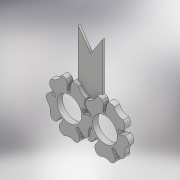
# Autodesk Inventor part: RosaV2
Saved by Autodesk Inventor 2017 (Build 210142000, 142)
## iProperties
Created: 2018-06-14
Part Number: RosaV2
Material: Generic
Document SubType Name: Modeling
Designer: Carolina Lema
Density: 1 g/cm^3
Appearance: Default
Author: Carolina Lema
Autodesk Inventor part; units mm, degrees
ref_plane "YZ Plane" through (0, 0, 0) normal (1, 0, 0) x (0, 1, 0)
ref_plane "XZ Plane" through (0, 0, 0) normal (0, 1, 0) x (-1, 0, 0)
ref_plane "XY Plane" through (0, 0, 0) normal (0, 0, 1) x (1, 0, 0)
sketch "Sketch1" plane through (0, 0, 0) normal (0, 1, 0) x (-1, 0, 0)
  arc A0 (-50.2935, -141.9625) -> (-50.5085, -138.2118) centre (-57.4787, -140.493) ccw
  arc A1 (-49.4604, -134.8668) -> (-50.5085, -138.2118) centre (-45.5145, -137.94) ccw
  arc A2 (-52.2706, -141.9093) -> (-53.5294, -134.3132) centre (-66.0628, -140.2926) ccw
  arc A3 (-60.8507, -147.4866) -> (-64.2809, -146.6761) centre (-66.0428, -161.7965) ccw
  circle A4 centre (-51.5636, -152.3854) radius 9
  arc A5 (-45.2271, -160.758) -> (-42.1345, -164.9104) centre (-15.6123, -141.9291) ccw
  arc A6 (-38.966, -164.9101) -> (-37.6707, -160.6686) centre (-43.0606, -161.3412) ccw
  arc A7 (-44.5421, -165.2935) -> (-46.8275, -161.7567) centre (-172.1244, -245.2288) ccw
  arc A8 (-37.8657, -145.4277) -> (-38.2191, -140.1494) centre (-41.6996, -143.0334) ccw
  arc A9 (-45.6096, -134.3885) -> (-38.2191, -140.1494) centre (-36.6467, -130.5112) ccw
  arc A10 (-36.1368, -156.274) -> (-37.6707, -160.6686) centre (-32.4682, -160.0194) ccw
  arc A11 (-36.1368, -156.274) -> (-34.6048, -152.385) centre (-42.1305, -151.6666) ccw
  arc A12 (-41.3682, -149.8747) -> (-38.503, -148.5121) centre (-47.6774, -132.9147) ccw
  arc A13 (-41.9398, -148.1863) -> (-37.8657, -145.4277) centre (-47.8277, -135.103) ccw
  arc A14 (-34.6048, -152.385) -> (-38.503, -148.5121) centre (-40.8573, -154.78) ccw
  arc A15 (-63.8657, -139.5775) -> (-58.174, -134.8668) centre (-65.1246, -132.2626) ccw
  arc A16 (-53.5294, -134.3132) -> (-58.174, -134.8668) centre (-55.4761, -137.7415) ccw
  arc A17 (-45.6096, -134.3885) -> (-49.4604, -134.8668) centre (-47.2959, -136.5525) ccw
  line L0 (-46.3394, -171.0352) -> (-46.3407, -171.0345)
  arc A18 (-48.8902, -170.6862) -> (-44.9412, -169.507) centre (-47.5666, -167.9168) ccw
  arc A19 (-65.6657, -161.3497) -> (-62.9245, -164.9101) centre (-62.7518, -161.9418) ccw
  arc A20 (-62.9245, -164.9101) -> (-58.2423, -160.4876) centre (-68.2851, -154.5449) ccw
  arc A21 (-56.5584, -161.6213) -> (-58.6246, -165.2834) centre (21.5695, -208.1162) ccw
  arc A22 (-58.6246, -165.2834) -> (-59.26, -166.6979) centre (-55.3426, -167.6077) ccw
  arc A23 (-59.26, -166.6979) -> (-53.816, -170.3276) centre (-55.8552, -167.4887) ccw
  arc A24 (-48.8902, -170.6862) -> (-53.816, -170.3276) centre (-51.7693, -176.2225) ccw
  arc A25 (-65.6657, -161.3497) -> (-67.4979, -155.3741) centre (-72.0774, -160.047) ccw
  arc A26 (-61.8781, -150.4206) -> (-66.2243, -148.9882) centre (-82.2432, -204.906) ccw
  arc A27 (-42.1345, -164.9104) -> (-38.966, -164.9101) centre (-40.5505, -161.8463) ccw
  arc A28 (-44.9412, -169.507) -> (-44.5421, -165.2935) centre (-48.2055, -167.0721) ccw
  arc A29 (-76.2935, -141.9625) -> (-76.5085, -138.2118) centre (-83.4787, -140.493) ccw
  arc A30 (-75.4604, -134.8668) -> (-76.5085, -138.2118) centre (-71.5145, -137.94) ccw
  arc A31 (-78.2706, -141.9093) -> (-79.5294, -134.3132) centre (-92.0628, -140.2926) ccw
  arc A32 (-86.8507, -147.4866) -> (-90.2809, -146.6761) centre (-92.0428, -161.7965) ccw
  circle A33 centre (-77.5636, -152.3854) radius 9
  arc A34 (-71.2271, -160.758) -> (-68.1345, -164.9104) centre (-41.6123, -141.9291) ccw
  arc A35 (-70.5421, -165.2935) -> (-72.8275, -161.7567) centre (-198.1244, -245.2288) ccw
  arc A36 (-63.8657, -145.4277) -> (-64.2191, -140.1494) centre (-67.6996, -143.0334) ccw
  arc A37 (-71.6096, -134.3885) -> (-64.2191, -140.1494) centre (-62.6467, -130.5112) ccw
  arc A38 (-67.9398, -148.1863) -> (-63.8657, -145.4277) centre (-73.8277, -135.103) ccw
  arc A39 (-90.7671, -139.6764) -> (-84.174, -134.8668) centre (-91.1246, -132.2626) ccw
  arc A40 (-79.5294, -134.3132) -> (-84.174, -134.8668) centre (-81.4761, -137.7415) ccw
  arc A41 (-71.6096, -134.3885) -> (-75.4604, -134.8668) centre (-73.2959, -136.5525) ccw
  line L1 (-72.3394, -171.0352) -> (-72.3407, -171.0345)
  arc A42 (-74.8902, -170.6862) -> (-70.9412, -169.507) centre (-73.5666, -167.9168) ccw
  arc A43 (-91.6657, -161.3497) -> (-88.9245, -164.9101) centre (-88.7518, -161.9418) ccw
  arc A44 (-88.9245, -164.9101) -> (-84.2423, -160.4876) centre (-94.2851, -154.5449) ccw
  arc A45 (-82.5584, -161.6213) -> (-84.6246, -165.2834) centre (-4.4305, -208.1162) ccw
  arc A46 (-84.6246, -165.2834) -> (-85.26, -166.6979) centre (-81.3426, -167.6077) ccw
  arc A47 (-85.26, -166.6979) -> (-79.816, -170.3276) centre (-81.8552, -167.4887) ccw
  arc A48 (-74.8902, -170.6862) -> (-79.816, -170.3276) centre (-77.7693, -176.2225) ccw
  arc A49 (-91.6639, -144.9966) -> (-90.2809, -146.6761) centre (-87.4857, -142.9652) ccw
  arc A50 (-90.7671, -139.6764) -> (-91.6639, -144.9966) centre (-87.4857, -142.9652) ccw
  arc A51 (-91.6657, -161.3497) -> (-94.028, -154.908) centre (-98.0774, -160.047) ccw
  arc A52 (-92.2243, -148.9882) -> (-94.028, -154.908) centre (-90.5316, -152.7386) ccw
  arc A53 (-87.8781, -150.4206) -> (-92.2243, -148.9882) centre (-108.2432, -204.906) ccw
  arc A54 (-68.1345, -164.9104) -> (-64.966, -164.9101) centre (-66.5505, -161.8463) ccw
  arc A55 (-70.9412, -169.507) -> (-70.5421, -165.2935) centre (-74.2055, -167.0721) ccw
  arc A56 (-66.2243, -148.9882) -> (-67.3918, -149.7806) centre (-64.5316, -152.7386) ccw
  circle A57 centre (-51.5636, -152.3854) radius 10.5
  circle A58 centre (-77.5636, -152.3854) radius 10.5
  arc A59 (-66.5505, -161.8463) -> (-64.966, -164.9101) centre (-62.3299, -161.6052) ccw
  arc A60 (-66.5505, -161.8463) -> (-67.9398, -156.5846) centre (-74.2403, -161.0624) ccw
  arc A61 (-64.2809, -146.6761) -> (-63.8657, -139.5775) centre (-67.8597, -142.9054) ccw
  line L2 (-53.5294, -134.3132) -> (-53.5294, -99.3132)
  line L3 (-53.5294, -99.3132) -> (-75.4604, -134.8668)
  line L4 (-75.4604, -134.8668) -> (-75.4604, -99.3132)
  line L5 (-75.4604, -99.3132) -> (-53.5294, -134.3132)
  point P0 (0, 0)
  point P1 (-51.4803, -152.4063)
  point P2 (-45.3977, -162.821)
  point P3 (-45.3977, -141.9574)
  point P4 (-33.5868, -132.2626)
  point P5 (-34.505, -161.7965)
  point P6 (-36.7472, -154.5449)
  point P7 (-47.2742, -170.9723)
  point P8 (-57.8397, -162.8189)
  point P9 (-56.1478, -170.9718)
  point P10 (-71.3977, -162.821)
  point P11 (-71.3977, -141.9574)
  point P12 (-59.5868, -132.2626)
  point P13 (-60.505, -161.7965)
  point P14 (-62.7472, -154.5449)
  point P15 (-73.2742, -170.9723)
  point P16 (-83.8397, -162.8189)
  point P17 (-82.1478, -170.9718)
  dimension "d2" = 21
  dimension "d3" = 21
  dimension "d0" = 18
  dimension "d1" = 18
  dimension "d6" = 35
  constraints: 128 point on circle, 60 centre point, 12 end point, 7 tangent, 2 coincident, 2 vertical, 1 concentric, 26 other
  measures "d0" diameter of A4
  measures "d1" diameter of A33
  measures "d6" distance of L2.start L2.end
extrude "Extrusion1" add sketch "Sketch1" along normal blind 4 contours A0 A1 A17 A9 A8 A13 A57 | A57 | A57 A3 A61 A15 A16 A2 | A12 A14 A11 A10 A6 A27 A5 A57 | A57 A20 A19 A25 A58 A56 A26 | A41 A37 A36 A38 A58 A29 A30 | A7 A28 A18 A24 A23 A22 A21 A57 | A58 | A58 A32 A49 A50 A39 A40 A31 | A60 A59 A54 A34 A58 | A58 A44 A43 A51 A52 A53 | A35 A55 A42 A48 A47 A46 A45 A58
sketch "Sketch3" plane through (0, 4, 0) normal (0, 1, 0) x (1, 0, 0)
  arc A0 (53.5294, 134.3132) -> (58.174, 134.8668) centre (55.4761, 137.7415) ccw projected
  line L0 (55.4761, 133.799) -> (55.4761, 98.799)
  arc A1 (71.6096, 134.3885) -> (75.4604, 134.8668) centre (73.2959, 136.5525) ccw projected
  line L1 (73.2959, 133.8091) -> (73.2959, 98.8091)
  line L2 (55.4761, 133.799) -> (61.5958, 151.1662)
  line L3 (61.5958, 151.1662) -> (68.0809, 150.5767)
  line L4 (68.0809, 150.5767) -> (73.2959, 133.8091)
  line L5 (55.4761, 98.799) -> (64.5905, 112.1825)
  line L6 (64.5905, 112.1825) -> (73.2959, 98.8091)
  point P0 (0, 0)
  dimension "d7" = 35
  dimension "d8" = 35
  constraints: 14 end point, 2 point on circle, 2 vertical
  measures "d7" distance of L0.start L0.end
  measures "d8" distance of L1.start L1.end
extrude "Extrusion2" add sketch "Sketch3" against normal blind 1.5
body "Solid1"
